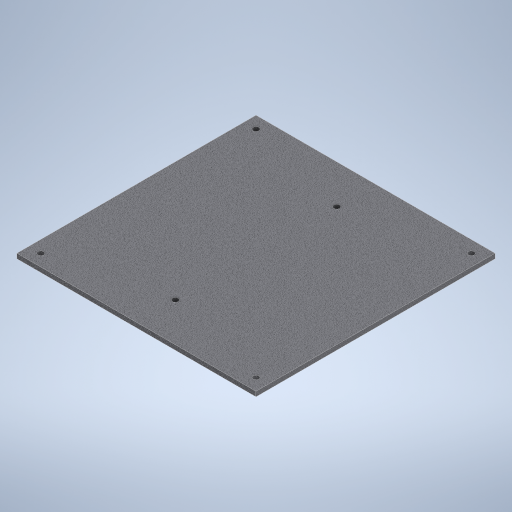
# Autodesk Inventor part: Mesa 1
Saved by Autodesk Inventor 2023.2 (Build 272271030, 271C)
## iProperties
Created: 2023-03-21
Part Number: Mesa 1
Material: Aço inoxidável
Document SubType Name: Sheet Metal
Designer: Mateus
Density: 8 g/cm^3
Sheet Metal Rule: Padrão_mm
Appearance: Ferro - Fundido
Mass: 1592.93 g
Surface Area: 843.534 cm^2
Volume: 199.116 cm^3
Author: Mateus
Autodesk Inventor part; units mm, degrees
ref_plane "YZ Plane" through (0, 0, 0) normal (1, 0, 0) x (0, 1, 0)
ref_plane "XZ Plane" through (0, 0, 0) normal (0, 1, 0) x (-1, 0, 0)
ref_plane "XY Plane" through (0, 0, 0) normal (0, 0, 1) x (1, 0, 0)
sketch "Esboço1" plane through (0, 0, 0) normal (0, 1, 0) x (-1, 0, 0)
  line L0 (0, 0) -> (200, 0)
  line L1 (200, 0) -> (200, -200)
  line L2 (200, -200) -> (0, -200)
  line L3 (0, -200) -> (0, 0)
  dimension "d0" = 200
  dimension "d1" = 200
  constraints: 8 end point, 2 parallel, 1 horizontal, 1 perpendicular
  measures "d0" distance of L1.end L2.end
  measures "d1" distance of L0.end L1.end
extrude "Extrusão1" add sketch "Esboço1" along normal blind 4
sketch "Esboço2" plane through (0, 4, 0) normal (0, 1, 0) x (1, 0, 0)
  line L0 (0, 0) -> (0, 200) projected
  line L1 (-200, 0) -> (0, 0) projected
  line L2 (-200, 200) -> (-200, 0) projected
  line L3 (0, 200) -> (-200, 200) projected
  point P0 (-10, 10)
  point P1 (-190, 10)
  point P2 (-190, 190)
  point P3 (-10, 190)
  dimension "d4" = 10
  dimension "d5" = 10
  dimension "d6" = 10
  dimension "d7" = 10
  dimension "d8" = 10
  dimension "d9" = 10
  dimension "d10" = 10
  dimension "d11" = 10
  dimension "d34" = 200
  dimension "d35" = 200
  measures "d4" distance from line of L0 point (-10, 10)
  measures "d5" distance from line of L1 point (-10, 10)
  measures "d6" distance from line of L0 point (-10, 190)
  measures "d7" distance from line of L2 point (-190, 10)
  measures "d8" distance from line of L2 point (-190, 190)
  measures "d9" distance from line of L1 point (-190, 10)
  measures "d10" distance from line of L3 point (-10, 190)
  measures "d11" distance from line of L3 point (-190, 190)
  measures "d34" distance of L0.start L0.end
  measures "d35" distance of L1.start L0.start
hole "Furo1" at (-10, 4, -10) at (-190, 4, -10) at (-190, 4, -190) at (-10, 4, -190) direction (0, -1, 0) diameter 5 end through all
sketch "Esboço3" plane through (0, 4, 0) normal (0, 1, 0) x (1, 0, 0)
  line L0 (-200, 200) -> (-200, 0) projected
  line L1 (-200, 0) -> (0, 0) projected
  line L2 (0, 0) -> (0, 200) projected
  line L3 (0, 200) -> (-200, 200) projected
  point P0 (-100, 32.5)
  point P1 (-100, 167.5)
  dimension "d19" = 100
  dimension "d22" = 0
  dimension "d46" = 200
  dimension "d47" = 135
  dimension "d48" = 32.5
  measures "d19" distance from line of L0 point (-100, 32.5)
  measures "d22" horizontal distance of point (-100, 32.5) point (-100, 167.5)
  measures "d46" distance of L2.end L0.start
  measures "d47" distance of point (-100, 32.5) point (-100, 167.5)
  measures "d48" distance from line of L1 point (-100, 32.5)
hole "Furo2" at (-100, 4, -32.5) at (-100, 4, -167.5) direction (0, -1, 0) diameter 5 depth 4 tip angle 118
equation "\"d5\" = d4"
equation "\"d6\" = d4"
equation "\"d7\" = d5"
equation "\"d8\" = d5"
equation "\"d9\" = d5"
equation "\"d10\" = d9"
equation "\"d11\" = d10"
equation "\"d17\" = Espessura"
equation "\"d19\" = 0.5 * d46"
equation "\"d48\" = -0.5 * d47 + 0.5 * d46"
equation "\"d32\" = Espessura"
equation "\"Raio_vergadura\" = Espessura"
equation "\"Largura_alívio_de_vergadura\" = Espessura"
equation "\"Profundidade_alívio_de_vergadura\" = 0.5 * Espessura"
equation "\"Tamanho_alívio_de_dobra\" = 4 * Espessura"
equation "\"Remanescente_mínimo\" = 2 * Espessura"
equation "\"Raiodetransição\" = Raio_vergadura"
equation "\"Tamanho_de_raio_de_Jacobi\" = Raio_vergadura"
equation "\"TamanhoFolga\" = Espessura"
equation "\"Espessura\" = 0.5"
